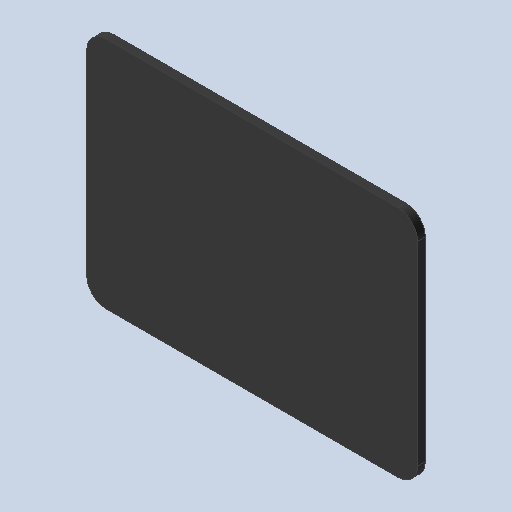
# Autodesk Inventor part: GBK-RK-0820 ring plate
Saved by Autodesk Inventor 2026 (Build 300175000, 175)
## iProperties
Created: 2024-05-23
Part Number: GBK-RK-0820 ring plate
Material: Generic
Document SubType Name: Sheet Metal
Designer: admin
Mass: 0.559799 g
Surface Area: 23.3947 cm^2
Volume: 0.559799 cm^3
Density: 1 g/cm^3
Flat Pattern Width: 12 cm
Flat Pattern Length: 17 cm
Flat Pattern Area: 204 cm^2
Sheet Metal Rule: По умолчанию_мм
Sheet Metal Width: 120,000 mm
Sheet Metal Length: 170,000 mm
Sheet Metal Area: 20400,000 mm^2
Appearance: Default
Author: admin
Autodesk Inventor part; units mm, degrees
ref_plane "YZ Plane" through (0, 0, 0) normal (1, 0, 0) x (0, 1, 0)
ref_plane "XZ Plane" through (0, 0, 0) normal (0, 1, 0) x (-1, 0, 0)
ref_plane "XY Plane" through (0, 0, 0) normal (0, 0, 1) x (1, 0, 0)
sketch "Sketch1" plane through (0, 0, 0) normal (0, 0, 1) x (1, 0, 0)
  line L0 (-85, 60) -> (85, 60)
  line L1 (85, 60) -> (85, -60)
  line L2 (85, -60) -> (-85, -60)
  line L3 (-85, -60) -> (-85, 60)
  line L4 (-85, 60) -> (85, -60) construction
  line L5 (85, 60) -> (-85, -60) construction
  line L6 (0, 60) -> (0, -60) construction
  point P0 (0, 0)
  dimension "d0" = 170
  dimension "d1" = 120
  measures "d0" distance of L1.end L2.end
  measures "d1" distance of L0.end L1.end
extrude "Plate1" add sketch "Sketch1" along normal blind 4
fillet "Corner Round1" radius 10 4 edges at (85, -60, 2) (85, 60, 2) (-85, -60, 2) (-85, 60, 2)
equation "\"d2\" = Thickness"
equation "\"BendRadius\" = Thickness"
equation "\"BendReliefWidth\" = Thickness"
equation "\"BendReliefDepth\" = 0.5 * Thickness"
equation "\"CornerReliefSize\" = 4 * Thickness"
equation "\"MinimumRemnant\" = 2 * Thickness"
equation "\"TransitionRadius\" = BendRadius"
equation "\"JacobiRadiusSize\" = BendRadius"
equation "\"GapSize\" = Thickness"
equation "\"Thickness\" = 4"
body "Solid1"
